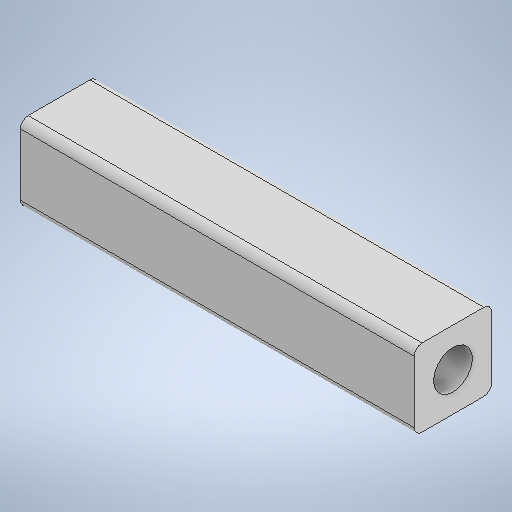
# Autodesk Inventor part: Contenedor
Saved by Autodesk Inventor 2025.1 (Build 291241000, 241)
## iProperties
Created: 2025-02-26
Part Number: Contenedor
Material: Generic
Document SubType Name: Modeling
Designer: yovan
Density: 1 g/cm^3
Appearance: Default
Author: yovan
Autodesk Inventor part; units mm, degrees
ref_plane "YZ Plane" through (0, 0, 0) normal (1, 0, 0) x (0, 1, 0)
ref_plane "XZ Plane" through (0, 0, 0) normal (0, 1, 0) x (-1, 0, 0)
ref_plane "XY Plane" through (0, 0, 0) normal (0, 0, 1) x (1, 0, 0)
sketch "Sketch1" plane through (0, 0, 0) normal (1, 0, 0) x (0, 1, 0)
  line L0 (0, 0) -> (100, 0)
  line L1 (100, 0) -> (100, -100)
  line L2 (100, -100) -> (0, -100)
  line L3 (0, -100) -> (0, 0)
  circle A0 centre (50, -50) radius 25
  line L4 (50, 0) -> (50, -50)
  line L5 (50, -50) -> (0, -50)
  dimension "d0" = 100
  dimension "d1" = 100
  dimension "d4" = 50
  dimension "d8" = 50
  dimension "d9" = 50
  constraints: 12 end point, 2 midpoint, 2 parallel, 2 perpendicular, 1 centre point, 1 horizontal, 1 vertical
  measures "d0" distance of L1.end L2.end
  measures "d1" distance of L0.end L1.end
  measures "d4" diameter of A0
  measures "d8" distance of L4.start L4.end
  measures "d9" distance of L4.end L5.end
extrude "Extrusion1" add sketch "Sketch1" along normal blind 500 contours L0 L4 A0 L5 L3 | L0 L1 L2 L3 L5 A0 L4
extrude "Extrusion2" add sketch "Sketch1" against normal blind 10
fillet "Fillet1" radius 10 4 edges at (245, 100, 0) (245, 0, 0) (245, 0, -100) (245, 100, -100)
body "Solid1"
